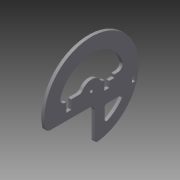
# Autodesk Inventor part: EChasisSide2
Saved by Autodesk Inventor 2015 (Build 190159000, 159)
## iProperties
Created: 2014-05-11
Part Number: EChasisSide2
Material: Generic
Document SubType Name: Modeling
Designer: STACKPOLE
Density: 1 g/cm^3
Appearance: Default
Author: STACKPOLE
Autodesk Inventor part; units mm, degrees
ref_plane "YZ Plane" through (0, 0, 0) normal (1, 0, 0) x (0, 1, 0)
ref_plane "XZ Plane" through (0, 0, 0) normal (0, 1, 0) x (-1, 0, 0)
ref_plane "XY Plane" through (0, 0, 0) normal (0, 0, 1) x (1, 0, 0)
sketch "Sketch1" plane through (0, 0, 0) normal (1, 0, 0) x (0, 1, 0)
  line L0 (-40.7216, -13) -> (-2, -13)
  arc A0 (30.5631, 9.4815) -> (-30.5631, 9.4815) centre (0, 0) ccw
  arc A1 (8.4591, 5.3333) -> (-8.4591, 5.3333) centre (0, 0) ccw
  circle A2 centre (0, 0) radius 1.5
  line L1 (3, -18) -> (3, -43.0842)
  arc A3 (3, -18) -> (-2, -13) centre (-2, -18) ccw
  arc A4 (6.4138, -46.0555) -> (-45.6278, -8.9639) centre (0, 0) ccw
  line L2 (-12.6886, 3) -> (-25.7876, 3)
  line L3 (12.6886, 3) -> (25.7876, 3)
  arc A5 (-30.5631, 9.4815) -> (-25.7876, 3) centre (-25.7876, 8) ccw
  arc A6 (-12.6886, 3) -> (-8.4591, 5.3333) centre (-12.6886, 8) ccw
  arc A7 (8.4591, 5.3333) -> (12.6886, 3) centre (12.6886, 8) ccw
  arc A8 (25.7876, 3) -> (30.5631, 9.4815) centre (25.7876, 8) ccw
  arc A9 (-45.6278, -8.9639) -> (-40.7216, -13) centre (-40.7216, -8) ccw
  arc A10 (3, -43.0842) -> (6.4138, -46.0555) centre (6, -43.0842) ccw
  point P0 (-44.6458, -13)
  point P1 (3, -13)
  point P2 (-10, 0)
  point P3 (10, 0)
  point P4 (-9.5394, 3)
  point P5 (9.5394, 3)
  point P6 (3, -31.881)
  point P7 (3, -46.4031)
  point P8 (-31.8591, 3)
  point P9 (31.8591, 3)
  dimension "d5" = 32
  dimension "d6" = 20
  dimension "d7" = 3
  dimension "d52" = 3
  dimension "d53" = 3
  dimension "d54" = 5
  dimension "d66" = 46.5
  dimension "d78" = 16
  dimension "d79" = 5
  dimension "d80" = 3
  dimension "d81" = 3
  dimension "d82" = 5
  constraints: 28 point on circle, 14 tangent, 11 centre point, 9 point on line, 8 end point, 4 coincident, 3 equal radius, 1 collinear, 1 horizontal, 1 perpendicular
  measures "d5" radius of A0
  measures "d6" diameter of A1
  measures "d7" diameter of A2
  measures "d52" distance from line of A4.centre L2
  measures "d53" distance from line of point (0, 0) L3
  measures "d54" radius of A5
  measures "d66" radius of A4
  measures "d78" distance between parallel lines of L2 L0
  measures "d79" radius of A9
  measures "d80" distance from line of L1 point (0, 0)
  measures "d81" radius of A10
  measures "d82" radius of A3
extrude "Extrusion3" add sketch "Sketch1" along normal blind 3
sketch "Sketch2" plane through (3, 0, 0) normal (1, 0, 0) x (0, 0, -1)
  arc A0 (-9.4815, 30.5631) -> (-9.4815, -30.5631) centre (0, 0) ccw projected
  line L0 (8, 43) -> (13, 43)
  line L1 (13, 43) -> (13, 40)
  line L2 (13, 40) -> (8, 40)
  line L3 (8, 40) -> (8, 43)
  dimension "d38" = 3
  dimension "d41" = 40
  dimension "d42" = 8
  dimension "d43" = 5
  constraints: 8 end point, 2 parallel, 1 horizontal, 1 perpendicular
  measures "d38" distance of L0.end L1.end
  measures "d41" distance from line of A0.centre L2
  measures "d42" distance from line of A0.centre L3
  measures "d43" distance of L0.start L0.end
extrude "Extrusion5" cut sketch "Sketch2" against normal through all
sketch "Sketch4" plane through (3, 0, 0) normal (1, 0, 0) x (0, 0, -1)
  arc A0 (-9.4815, 30.5631) -> (-9.4815, -30.5631) centre (0, 0) ccw projected
  line L0 (-3, 25.7876) -> (-3, 12.6886) projected
  line L1 (-3, -12.6886) -> (-3, -25.7876) projected
  line L2 (-3, -20) -> (6, -20)
  line L3 (6, -20) -> (6, -25)
  line L4 (6, -25) -> (-3, -25)
  line L5 (-3, -25) -> (-3, -20)
  line L6 (-3, 17.5) -> (6, 17.5)
  line L7 (6, 17.5) -> (6, 12.5)
  line L8 (6, 12.5) -> (-3, 12.5)
  line L9 (-3, 12.5) -> (-3, 17.5)
  dimension "d57" = 9
  dimension "d59" = 5
  dimension "d60" = 20
  dimension "d61" = 9
  dimension "d62" = 5
  dimension "d63" = 12.5
  constraints: 16 end point, 4 parallel, 2 horizontal, 2 perpendicular, 2 point on line
  measures "d57" distance of L3.end L4.end
  measures "d59" distance of L2.end L3.end
  measures "d60" distance from line of A0.centre L2
  measures "d61" distance of L6.start L6.end
  measures "d62" distance of L6.end L7.end
  measures "d63" distance from line of A0.centre L8
extrude "Extrusion6" cut sketch "Sketch4" against normal through all
sketch "Sketch5" plane through (3, 0, 0) normal (1, 0, 0) x (0, 0, -1)
  line L0 (-3, 17.5) -> (0, 17.5)
  line L1 (0, 17.5) -> (0, 22.5)
  line L2 (0, 22.5) -> (-3, 22.5)
  line L3 (-3, 22.5) -> (-3, 17.5)
  point P0 (0, 0)
  dimension "d67" = 5
  dimension "d68" = 3
  constraints: 8 end point, 2 parallel, 1 horizontal, 1 perpendicular
  measures "d67" distance of L0.end L1.end
  measures "d68" distance of L1.end L2.end
extrude "Extrusion7" cut sketch "Sketch5" against normal through all
sketch "Sketch6" plane through (3, 0, 0) normal (1, 0, 0) x (0, 0, -1)
  circle A0 centre (0, 0) radius 1.5 projected
  arc A1 (32.8695, 15.8696) -> (21.1594, 29.741) centre (0, 0) ccw
  line L0 (31.0685, 13) -> (20, 13)
  line L1 (18, 15) -> (18, 28.1114)
  line L2 (18, 3) -> (43.0842, 3) projected
  line L3 (13, -40.7216) -> (13, -2) projected
  arc A2 (31.0685, 13) -> (32.8695, 15.8696) centre (31.0685, 15) ccw
  arc A3 (21.1594, 29.741) -> (18, 28.1114) centre (20, 28.1114) ccw
  arc A4 (18, 15) -> (20, 13) centre (20, 15) ccw
  point P0 (41.1696, 0.4856)
  point P1 (14.881, -40.3065)
  point P2 (14.881, -4.5144)
  point P3 (18, 31.753)
  point P4 (34.1065, 13)
  point P5 (43.0842, 3)
  point P6 (13, -2)
  dimension "d72" = 73
  dimension "d73" = 10
  dimension "d74" = 5
  dimension "d75" = 2
  constraints: 10 point on circle, 6 tangent, 4 centre point, 4 end point, 2 equal radius, 2 point on line, 1 coincident, 1 horizontal, 1 perpendicular, 2 other
  measures "d72" diameter of A1
  measures "d75" radius of A2
extrude "Extrusion8" cut sketch "Sketch6" against normal through all contours A2 L0 A4 L1 A3 A1
body "Solid3"
